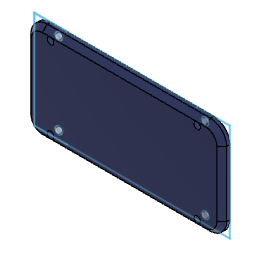
right lid (Autodesk Fusion 360 design; units mm, degrees)
Autodesk Fusion 360 part; units mm, degrees
sketch "sketch 427" plane through (0, 71.5775, 0) normal (0, -1, 0) x (1, 0, 0)
  circle A0 centre (46.5972, 163.8238) radius 2
  circle A1 centre (46.5972, 163.8238) radius 2
  circle A2 centre (136.5972, 113.8238) radius 2
  circle A3 centre (46.5972, 113.8238) radius 2
  circle A4 centre (46.5972, 113.8238) radius 2
  circle A5 centre (136.5972, 163.8238) radius 2
  line L0 (151.5972, 168.8238) -> (131.5972, 168.8238)
  line L1 (51.5972, 168.8238) -> (131.5972, 168.8238)
  line L2 (31.5972, 168.8238) -> (51.5972, 168.8238)
  line L3 (31.5972, 168.8238) -> (51.5972, 168.8238)
  line L4 (31.5972, 168.8238) -> (31.5972, 108.8238)
  line L5 (31.5972, 168.8238) -> (31.5972, 108.8238)
  line L6 (31.5972, 108.8238) -> (51.5972, 108.8238)
  line L7 (31.5972, 108.8238) -> (51.5972, 108.8238)
  line L8 (51.5972, 108.8238) -> (131.5972, 108.8238)
  line L9 (151.5972, 108.8238) -> (131.5972, 108.8238)
  line L10 (151.5972, 168.8238) -> (151.5972, 108.8238)
extrude "Extrude1" add sketch "sketch 427" along normal blind 5
fillet "Fillet1" radius 10 4 edges at (31.5972, 69.0775, 168.8238) (151.5972, 69.0775, 168.8238) (151.5972, 69.0775, 108.8238) (31.5972, 69.0775, 108.8238)
chamfer "Chamfer1" distance 3 angle 45 10 edges at (91.5972, 66.5775, 168.8238) (34.5261, 66.5775, 165.8949) (31.5972, 66.5775, 138.8238) (34.5261, 66.5775, 111.7528) (46.5972, 66.5775, 108.8238) (91.5972, 66.5775, 108.8238) (136.5972, 66.5775, 108.8238) (148.6682, 66.5775, 111.7528) (151.5972, 66.5775, 138.8238) (148.6682, 66.5775, 165.8949)
